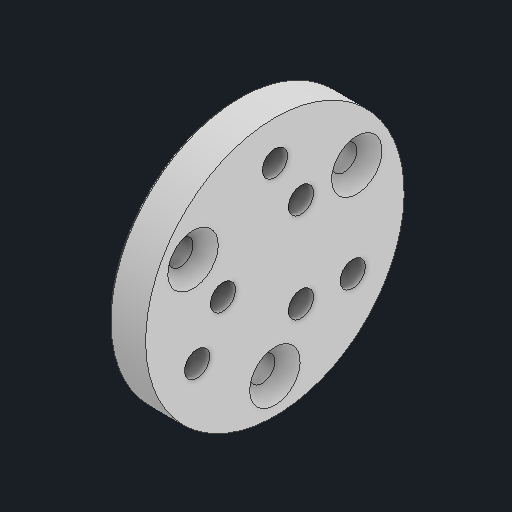
# Autodesk Inventor part: waist_hip_joint_v2
Saved by Autodesk Inventor 2026 (Build 300175000, 175)
## iProperties
Created: 2025-07-13
Part Number: waist_hip_joint_v2
Material: Generic
Document SubType Name: Modeling
Designer: User
Density: 1 g/cm^3
Appearance: Default
Author: User
Autodesk Inventor part; units mm, degrees
ref_plane "YZ Plane" through (0, 0, 0) normal (1, 0, 0) x (0, 1, 0)
ref_plane "XZ Plane" through (0, 0, 0) normal (0, 1, 0) x (-1, 0, 0)
ref_plane "XY Plane" through (0, 0, 0) normal (0, 0, 1) x (1, 0, 0)
sketch "Sketch1" plane through (0, 0, 0) normal (1, 0, 0) x (0, 1, 0)
  circle A0 centre (0, 0) radius 20.5
  circle A1 centre (0, 0) radius 15 construction
  line L0 (0, 0) -> (16.0369, -27.7767) construction
  line L1 (16.0369, -27.7767) -> (16.0369, 0) construction
  line L2 (16.0369, 0) -> (0, 0) construction
  circle A2 centre (0, 0) radius 14.25 construction
  line L3 (0, 0) -> (-15.2425, -26.4009) construction
  line L4 (-15.2425, -26.4009) -> (-20.5, 0) construction
  line L5 (0, 0) -> (-20.5, 0) construction
  circle A3 centre (7.5, -12.9904) radius 2
  circle A4 centre (7.5, 12.9904) radius 2
  circle A5 centre (-15, 0) radius 2
  circle A6 centre (14.25, 0) radius 2
  circle A7 centre (-7.125, 12.3409) radius 2
  circle A8 centre (-7.125, -12.3409) radius 2
  dimension "d0" = 41
  dimension "d1" = 30
  dimension "d16" = 28.5
  dimension "d15" = 60
  dimension "d22" = 60
  dimension "d28" = 4
  dimension "d31" = 360
  dimension "d33" = 4
  dimension "d36" = 360
  constraints: 12 end point, 6 centre point, 3 coincident, 2 horizontal alignment, 1 horizontal, 1 perpendicular, 1 point on line, 1 vertical, 21 other
  measures "d15" angle of L2 L0
  measures "d22" angle of L5 L3
  measures "d28" diameter of A3
  measures "d33" diameter of A6
extrude "Extrusion1" add sketch "Sketch1" along normal blind 6
chamfer "Chamfer2" distance 0.5 angle 45 1 edges at (0, -20.5, 0)
chamfer "Chamfer3" distance 2 angle 45 3 edges at (6, 5.5, 12.9904) (6, 5.5, -12.9904) (6, -17, 0)
sketch "Sketch5" plane through (6, 0, 0) normal (1, 0, 0) x (0, 0, -1)
  circle A0 centre (0, 0) radius 8.25 construction
  line L0 (0, 0) -> (16.9526, 0) construction
  line L1 (0, 0) -> (12.1845, 21.1041) construction
  circle A1 centre (4.125, 7.1447) radius 2
  circle A2 centre (-8.25, 0) radius 2
  circle A3 centre (4.125, -7.1447) radius 2
  dimension "d44" = 16.5
  dimension "d45" = 60
  dimension "d46" = 4
  dimension "d49" = 360
  constraints: 4 end point, 3 centre point, 1 coincident, 1 horizontal, 1 point on line, 10 other
  measures "d45" angle of L0 L1
  measures "d46" diameter of A1
extrude "Extrusion3" cut sketch "Sketch5" against normal blind 3
body "Solid1"
